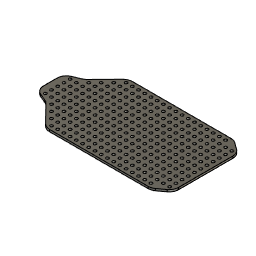
Base Plate (Autodesk Fusion 360 design; units mm, degrees)
Autodesk Fusion 360 part; units mm, degrees
sketch "Sketch1" plane through (0, 0, 0) normal (0, 0, 1) x (1, 0, 0)
  line L0 (-125, 0) -> (125, 0)
  line L1 (-125, 0) -> (-125, 21)
  line L2 (-125, 21) -> (-101, 31)
  line L3 (-101, 31) -> (-66, 66.7071)
  line L4 (-66, 66.7071) -> (104, 66.7071)
  line L5 (104, 66.7071) -> (125, 51.3774)
  line L6 (125, 51.3774) -> (125, 0)
  line L7 (-66, -66.7071) -> (104, -66.7071)
  line L8 (125, -51.3774) -> (125, 0)
  line L9 (-125, -21) -> (-101, -31)
  line L10 (104, -66.7071) -> (125, -51.3774)
  line L11 (-101, -31) -> (-66, -66.7071)
  line L12 (-125, 0) -> (-125, -21)
  line L13 (-125, 0) -> (125, 0) construction
  dimension "d1" = 250
  dimension "d2" = 21
  dimension "d3" = 26
  dimension "d4" = 24
  dimension "d5" = 50
  dimension "d6" = 35
  dimension "d7" = 170
  dimension "d8" = 26
  constraint horizontal L0
  constraint midpoint origin L0
  constraint perpendicular L0 L1
  constraint horizontal L4
  constraint symmetric L1.start L0 L12.start
  constraint symmetric L6.end L0 L8.end
  constraint symmetric L0 L1.end L9.start
  constraint symmetric L0 L2.end L9.end
  constraint symmetric L0 L3.end L7.start
  constraint symmetric L0 L4.end L7.end
  constraint symmetric L0 L5.end L8.start
  constraint vertical L6
  measures "d1" distance of L0.start L0.end
  measures "d2" distance of L0.start L1.end
  measures "d3" distance of L1.end L2.end
  measures "d4" horizontal distance of L1.end L2.end
  measures "d5" distance of L2.end L3.end
  measures "d6" horizontal distance of L2.end L3.end
  measures "d7" distance of L3.end L4.end
  measures "d8" distance of L4.end L5.end
extrude "Extrude1" add sketch "Sketch1" along normal blind 3.175
fillet "Fillet1" radius 15 10 edges at (-101, -31, 1.5875) (-125, -21, 1.5875) (-101, 31, 1.5875) (-125, 21, 1.5875) (-66, 66.7071, 1.5875) (-66, -66.7071, 1.5875) (104, -66.7071, 1.5875) (125, -51.3774, 1.5875) (125, 51.3774, 1.5875) (104, 66.7071, 1.5875)
sketch "Sketch2" plane through (0, 0, 3.175) normal (0, 0, 1) x (-1, 0, 0)
  arc A0 (-107.9516, -63.8225) -> (-99.1075, -66.7071) centre (-99.1075, -51.7071) ccw
  line L0 (-99.1075, -66.7071) -> (59.6987, -66.7071)
  arc A1 (59.6987, -66.7071) -> (70.4109, -62.2071) centre (59.6987, -51.7071) ccw
  line L1 (70.4109, -62.2071) -> (98.8682, -33.1748)
  arc A2 (103.8111, -29.8287) -> (98.8682, -33.1748) centre (109.5804, -43.6748) ccw
  line L2 (103.8111, -29.8287) -> (115.7692, -24.8462)
  arc A3 (115.7692, -24.8462) -> (125, -11) centre (110, -11) ccw
  line L3 (125, -11) -> (125, 11)
  arc A4 (125, 11) -> (115.7692, 24.8462) centre (110, 11) ccw
  line L4 (115.7692, 24.8462) -> (103.8111, 29.8287)
  arc A5 (98.8682, 33.1748) -> (103.8111, 29.8287) centre (109.5804, 43.6748) ccw
  line L5 (98.8682, 33.1748) -> (70.4109, 62.2071)
  arc A6 (70.4109, 62.2071) -> (59.6987, 66.7071) centre (59.6987, 51.7071) ccw
  line L6 (59.6987, 66.7071) -> (-99.1075, 66.7071)
  arc A7 (-99.1075, 66.7071) -> (-107.9516, 63.8225) centre (-99.1075, 51.7071) ccw
  line L7 (-107.9516, 63.8225) -> (-118.8441, 55.8712)
  arc A8 (-118.8441, 55.8712) -> (-125, 43.7558) centre (-110, 43.7558) ccw
  line L8 (-125, 43.7558) -> (-125, -43.7558)
  arc A9 (-125, -43.7558) -> (-118.8441, -55.8712) centre (-110, -43.7558) ccw
  line L9 (-118.8441, -55.8712) -> (-107.9516, -63.8225)
  circle A10 centre (-117, 0) radius 2.25
  line L10 (-125, 0) -> (125, 0) construction
  circle A11 centre (-117, 0) radius 2.25
  point P0 (-107, 0)
  point P1 (-97, 0)
  point P2 (-117, 10)
  point P3 (-107, 10)
  point P4 (-97, 10)
  point P5 (-117, 20)
  point P6 (-107, 20)
  point P7 (-97, 20)
  point P8 (-87, 0)
  point P9 (-77, 0)
  point P10 (-67, 0)
  point P11 (-57, 0)
  point P12 (-47, 0)
  point P13 (-37, 0)
  point P14 (-27, 0)
  point P15 (-17, 0)
  point P16 (-7, 0)
  point P17 (3, 0)
  point P18 (13, 0)
  point P19 (23, 0)
  point P20 (33, 0)
  point P21 (43, 0)
  point P22 (53, 0)
  point P23 (63, 0)
  point P24 (73, 0)
  point P25 (83, 0)
  point P26 (93, 0)
  point P27 (103, 0)
  point P28 (113, 0)
  point P29 (-87, 10)
  point P30 (-77, 10)
  point P31 (-67, 10)
  point P32 (-57, 10)
  point P33 (-47, 10)
  point P34 (-37, 10)
  point P35 (-27, 10)
  point P36 (-17, 10)
  point P37 (-7, 10)
  point P38 (3, 10)
  point P39 (13, 10)
  point P40 (23, 10)
  point P41 (33, 10)
  point P42 (43, 10)
  point P43 (53, 10)
  point P44 (63, 10)
  point P45 (73, 10)
  point P46 (83, 10)
  point P47 (93, 10)
  point P48 (103, 10)
  point P49 (113, 10)
  point P50 (-87, 20)
  point P51 (-77, 20)
  point P52 (-67, 20)
  point P53 (-57, 20)
  point P54 (-47, 20)
  point P55 (-37, 20)
  point P56 (-27, 20)
  point P57 (-17, 20)
  point P58 (-7, 20)
  point P59 (3, 20)
  point P60 (13, 20)
  point P61 (23, 20)
  point P62 (33, 20)
  point P63 (43, 20)
  point P64 (53, 20)
  point P65 (63, 20)
  point P66 (73, 20)
  point P67 (83, 20)
  point P68 (93, 20)
  point P69 (103, 20)
  point P70 (113, 20)
  point P71 (-117, 30)
  point P72 (-107, 30)
  point P73 (-97, 30)
  point P74 (-87, 30)
  point P75 (-77, 30)
  point P76 (-67, 30)
  point P77 (-57, 30)
  point P78 (-47, 30)
  point P79 (-37, 30)
  point P80 (-27, 30)
  point P81 (-17, 30)
  point P82 (-7, 30)
  point P83 (3, 30)
  point P84 (13, 30)
  point P85 (23, 30)
  point P86 (33, 30)
  point P87 (43, 30)
  point P88 (53, 30)
  point P89 (63, 30)
  point P90 (73, 30)
  point P91 (83, 30)
  point P92 (93, 30)
  point P93 (-117, 40)
  point P94 (-107, 40)
  point P95 (-97, 40)
  point P96 (-87, 40)
  point P97 (-77, 40)
  point P98 (-67, 40)
  point P99 (-57, 40)
  point P100 (-47, 40)
  point P101 (-37, 40)
  point P102 (-27, 40)
  point P103 (-17, 40)
  point P104 (-7, 40)
  point P105 (3, 40)
  point P106 (13, 40)
  point P107 (23, 40)
  point P108 (33, 40)
  point P109 (43, 40)
  point P110 (53, 40)
  point P111 (63, 40)
  point P112 (73, 40)
  point P113 (83, 40)
  point P114 (-117, 50)
  point P115 (-107, 50)
  point P116 (-97, 50)
  point P117 (-87, 50)
  point P118 (-77, 50)
  point P119 (-67, 50)
  point P120 (-57, 50)
  point P121 (-47, 50)
  point P122 (-37, 50)
  point P123 (-27, 50)
  point P124 (-17, 50)
  point P125 (-7, 50)
  point P126 (3, 50)
  point P127 (13, 50)
  point P128 (23, 50)
  point P129 (33, 50)
  point P130 (43, 50)
  point P131 (53, 50)
  point P132 (63, 50)
  point P133 (73, 50)
  point P134 (-97, 60)
  point P135 (-87, 60)
  point P136 (-77, 60)
  point P137 (-67, 60)
  point P138 (-57, 60)
  point P139 (-47, 60)
  point P140 (-37, 60)
  point P141 (-27, 60)
  point P142 (-17, 60)
  point P143 (-7, 60)
  point P144 (3, 60)
  point P145 (13, 60)
  point P146 (23, 60)
  point P147 (33, 60)
  point P148 (43, 60)
  point P149 (53, 60)
  point P150 (63, 60)
  point P151 (93, 0)
  point P152 (103, 0)
  point P153 (83, -10)
  point P154 (113, 0)
  point P155 (83, -20)
  point P156 (83, 0)
  point P157 (113, -10)
  point P158 (113, -20)
  point P159 (73, -20)
  point P160 (93, -10)
  point P161 (103, -20)
  point P162 (73, 0)
  point P163 (73, -10)
  point P164 (103, -10)
  point P165 (93, -20)
  point P166 (-67, -30)
  point P167 (-37, -40)
  point P168 (-47, -50)
  point P169 (-7, -10)
  point P170 (-117, -30)
  point P171 (3, -30)
  point P172 (-17, -50)
  point P173 (-47, -10)
  point P174 (-67, 0)
  point P175 (-107, -40)
  point P176 (-57, -40)
  point P177 (33, 0)
  point P178 (-107, -50)
  point P179 (-87, 0)
  point P180 (-117, -20)
  point P181 (-67, -50)
  point P182 (-57, -30)
  point P183 (-7, -50)
  point P184 (53, -30)
  point P185 (-47, -30)
  point P186 (-17, -40)
  point P187 (13, -10)
  point P188 (-107, -30)
  point P189 (-27, -20)
  point P190 (-77, -20)
  point P191 (-87, -10)
  point P192 (23, -20)
  point P193 (53, -20)
  point P194 (-47, -40)
  point P195 (-17, 0)
  point P196 (-27, -10)
  point P197 (-107, -10)
  point P198 (-27, -50)
  point P199 (-97, -40)
  point P200 (-37, -50)
  point P201 (-117, -10)
  point P202 (-7, -40)
  point P203 (63, -50)
  point P204 (63, -40)
  point P205 (-77, -30)
  point P206 (-87, -20)
  point P207 (-97, -20)
  point P208 (63, -10)
  point P209 (63, -30)
  point P210 (43, 0)
  point P211 (-7, -20)
  point P212 (3, 0)
  point P213 (63, -20)
  point P214 (63, 0)
  point P215 (-67, -20)
  point P216 (33, -30)
  point P217 (53, -10)
  point P218 (13, -40)
  point P219 (23, -30)
  point P220 (23, 0)
  point P221 (-87, -40)
  point P222 (-97, 0)
  point P223 (-107, 0)
  point P224 (-97, -30)
  point P225 (33, -20)
  point P226 (-107, -20)
  point P227 (-67, -10)
  point P228 (-77, 0)
  point P229 (-57, -50)
  point P230 (-7, -30)
  point P231 (-57, 0)
  point P232 (-77, -10)
  point P233 (-117, -50)
  point P234 (-27, -30)
  point P235 (-47, 0)
  point P236 (33, -10)
  point P237 (43, -20)
  point P238 (3, -10)
  point P239 (-97, -10)
  point P240 (53, -40)
  point P241 (23, -40)
  point P242 (33, -50)
  point P243 (23, -10)
  point P244 (43, -30)
  point P245 (3, -40)
  point P246 (-17, -10)
  point P247 (43, -40)
  point P248 (-77, -50)
  point P249 (-87, -50)
  point P250 (33, -40)
  point P251 (-27, 0)
  point P252 (13, -30)
  point P253 (-7, 0)
  point P254 (3, -50)
  point P255 (-77, -40)
  point P256 (-87, -30)
  point P257 (-17, -20)
  point P258 (13, -20)
  point P259 (-67, -40)
  point P260 (13, -50)
  point P261 (-27, -40)
  point P262 (-47, -20)
  point P263 (53, -50)
  point P264 (-97, -50)
  point P265 (23, -50)
  point P266 (-117, -40)
  point P267 (53, 0)
  point P268 (3, -20)
  point P269 (43, -50)
  point P270 (-37, -30)
  point P271 (13, 0)
  point P272 (43, -10)
  point P273 (-57, -10)
  point P274 (-57, -20)
  point P275 (-37, -10)
  point P276 (-37, 0)
  point P277 (-17, -30)
  point P278 (-37, -20)
  point P279 (73, -40)
  point P280 (83, -30)
  point P281 (73, -30)
  point P282 (73, -50)
  point P283 (83, -40)
  point P284 (93, -30)
  point P285 (-67, -60)
  point P286 (63, -60)
  point P287 (-17, -60)
  point P288 (13, -60)
  point P289 (43, -60)
  point P290 (-77, -60)
  point P291 (23, -60)
  point P292 (-97, -60)
  point P293 (3, -60)
  point P294 (33, -60)
  point P295 (-7, -60)
  point P296 (-57, -60)
  point P297 (-37, -60)
  point P298 (-27, -60)
  point P299 (-47, -60)
  point P300 (-87, -60)
  point P301 (53, -60)
  dimension "d14" = 4.5
  dimension "d15" = 8
  dimension "d18" = 10
  dimension "d19" = 10
  constraint midpoint L8 L10.start
  constraint midpoint L3 L10.end
  constraint symmetric A10 L10 A11
  constraint symmetric P223 L10 P0
  constraint symmetric P222 L10 P1
  constraint symmetric P2 L10 P201
  constraint symmetric P3 L10 P197
  constraint symmetric P4 L10 P239
  constraint symmetric P5 L10 P180
  constraint symmetric P6 L10 P226
  constraint symmetric P7 L10 P207
  constraint symmetric P179 L10 P8
  constraint symmetric P228 L10 P9
  constraint symmetric P174 L10 P10
  constraint symmetric P231 L10 P11
  constraint symmetric P235 L10 P12
  constraint symmetric P276 L10 P13
  constraint symmetric P251 L10 P14
  constraint symmetric P195 L10 P15
  constraint symmetric P253 L10 P16
  constraint symmetric P212 L10 P17
  constraint symmetric P271 L10 P18
  constraint symmetric P220 L10 P19
  constraint symmetric P177 L10 P20
  constraint symmetric P210 L10 P21
  constraint symmetric P267 L10 P22
  constraint symmetric P214 L10 P23
  constraint symmetric P162 L10 P24
  constraint symmetric P156 L10 P25
  constraint symmetric P151 L10 P26
  constraint symmetric P152 L10 P27
  constraint symmetric P154 L10 P28
  constraint symmetric P29 L10 P191
  constraint symmetric P30 L10 P232
  constraint symmetric P31 L10 P227
  constraint symmetric P32 L10 P273
  constraint symmetric P33 L10 P173
  constraint symmetric P34 L10 P275
  constraint symmetric P35 L10 P196
  constraint symmetric P36 L10 P246
  constraint symmetric P37 L10 P169
  constraint symmetric P38 L10 P238
  constraint symmetric P39 L10 P187
  constraint symmetric P40 L10 P243
  constraint symmetric P41 L10 P236
  constraint symmetric P42 L10 P272
  constraint symmetric P43 L10 P217
  constraint symmetric P44 L10 P208
  constraint symmetric P45 L10 P163
  constraint symmetric P46 L10 P153
  constraint symmetric P47 L10 P160
  constraint symmetric P48 L10 P164
  constraint symmetric P49 L10 P157
  constraint symmetric P50 L10 P206
  constraint symmetric P51 L10 P190
  constraint symmetric P52 L10 P215
  constraint symmetric P53 L10 P274
  constraint symmetric P54 L10 P262
  constraint symmetric P55 L10 P278
  constraint symmetric P56 L10 P189
  constraint symmetric P57 L10 P257
  constraint symmetric P58 L10 P211
  constraint symmetric P59 L10 P268
  constraint symmetric P60 L10 P258
  constraint symmetric P61 L10 P192
  constraint symmetric P62 L10 P225
  constraint symmetric P63 L10 P237
  constraint symmetric P64 L10 P193
  constraint symmetric P65 L10 P213
  constraint symmetric P66 L10 P159
  constraint symmetric P67 L10 P155
  constraint symmetric P68 L10 P165
  constraint symmetric P69 L10 P161
  constraint symmetric P70 L10 P158
  constraint symmetric P71 L10 P170
  constraint symmetric P72 L10 P188
  constraint symmetric P73 L10 P224
  constraint symmetric P74 L10 P256
  constraint symmetric P75 L10 P205
  constraint symmetric P76 L10 P166
  constraint symmetric P77 L10 P182
  constraint symmetric P78 L10 P185
  constraint symmetric P79 L10 P270
  constraint symmetric P80 L10 P234
  constraint symmetric P81 L10 P277
  constraint symmetric P82 L10 P230
  constraint symmetric P83 L10 P171
  constraint symmetric P84 L10 P252
  constraint symmetric P85 L10 P219
  constraint symmetric P86 L10 P216
  constraint symmetric P87 L10 P244
  constraint symmetric P88 L10 P184
  constraint symmetric P89 L10 P209
  constraint symmetric P90 L10 P281
  constraint symmetric P91 L10 P280
  constraint symmetric P92 L10 P284
  constraint symmetric P93 L10 P266
  constraint symmetric P94 L10 P175
  constraint symmetric P95 L10 P199
  constraint symmetric P96 L10 P221
  constraint symmetric P97 L10 P255
  constraint symmetric P98 L10 P259
  constraint symmetric P99 L10 P176
  constraint symmetric P100 L10 P194
  constraint symmetric P101 L10 P167
  constraint symmetric P102 L10 P261
  constraint symmetric P103 L10 P186
  constraint symmetric P104 L10 P202
  constraint symmetric P105 L10 P245
  constraint symmetric P106 L10 P218
  constraint symmetric P107 L10 P241
  constraint symmetric P108 L10 P250
  constraint symmetric P109 L10 P247
  constraint symmetric P110 L10 P240
  constraint symmetric P111 L10 P204
  constraint symmetric P112 L10 P279
  constraint symmetric P113 L10 P283
  constraint symmetric P114 L10 P233
  constraint symmetric P115 L10 P178
  constraint symmetric P116 L10 P264
  constraint symmetric P117 L10 P249
  constraint symmetric P118 L10 P248
  constraint symmetric P119 L10 P181
  constraint symmetric P120 L10 P229
  constraint symmetric P121 L10 P168
  constraint symmetric P122 L10 P200
  constraint symmetric P123 L10 P198
  constraint symmetric P124 L10 P172
  constraint symmetric P125 L10 P183
  constraint symmetric P126 L10 P254
  constraint symmetric P127 L10 P260
  constraint symmetric P128 L10 P265
  constraint symmetric P129 L10 P242
  constraint symmetric P130 L10 P269
  constraint symmetric P131 L10 P263
  constraint symmetric P132 L10 P203
  constraint symmetric P133 L10 P282
  constraint symmetric P134 L10 P292
  constraint symmetric P135 L10 P300
  constraint symmetric P136 L10 P290
  constraint symmetric P137 L10 P285
  constraint symmetric P138 L10 P296
  constraint symmetric P139 L10 P299
  constraint symmetric P140 L10 P297
  constraint symmetric P141 L10 P298
  constraint symmetric P142 L10 P287
  constraint symmetric P143 L10 P295
  constraint symmetric P144 L10 P293
  constraint symmetric P145 L10 P288
  constraint symmetric P146 L10 P291
  constraint symmetric P147 L10 P294
  constraint symmetric P148 L10 P289
  constraint symmetric P149 L10 P301
  constraint symmetric P150 L10 P286
  measures "d14" diameter of A10
  measures "d15" distance of L8 A10.centre
hole "Hole1" at (67, 20, 3.175) at (87, 50, 3.175) at (-43, -40, 3.175) at (17, 20, 3.175) at (-23, -50, 3.175) at (87, 30, 3.175) at (107, -40, 3.175) at (117, -50, 3.175) at (-13, -60, 3.175) at (-33, 20, 3.175) at (77, 40, 3.175) at (117, 20, 3.175) at (-73, -10, 3.175) at (47, 40, 3.175) at (-103, -20, 3.175) at (57, 30, 3.175) at (97, 50, 3.175) at (97, -50, 3.175) at (17, 30, 3.175) at (67, 40, 3.175) at (-53, 60, 3.175) at (67, -50, 3.175) at (-23, 50, 3.175) at (-53, -40, 3.175) at (97, 30, 3.175) at (97, 20, 3.175) at (57, 20, 3.175) at (117, 50, 3.175) at (-23, -60, 3.175) at (-83, -20, 3.175) at (27, 30, 3.175) at (-13, -50, 3.175) at (-43, 40, 3.175) at (-3, -50, 3.175) at (-3, -40, 3.175) at (87, 20, 3.175) at (77, 60, 3.175) at (-23, 40, 3.175) at (37, 30, 3.175) at (-73, -30, 3.175) at (-73, 20, 3.175) at (-113, 20, 3.175) at (77, -60, 3.175) at (47, 30, 3.175) at (97, -60, 3.175) at (77, -50, 3.175) at (77, 30, 3.175) at (-103, 0, 3.175) at (97, 40, 3.175) at (67, -60, 3.175) at (-93, 30, 3.175) at (7, 20, 3.175) at (-83, 30, 3.175) at (117, -40, 3.175) at (-43, -60, 3.175) at (7, 0, 3.175) at (107, -10, 3.175) at (7, -20, 3.175) at (57, -60, 3.175) at (7, -50, 3.175) at (117, 10, 3.175) at (117, 0, 3.175) at (37, -30, 3.175) at (-43, -30, 3.175) at (7, -60, 3.175) at (-3, 0, 3.175) at (-53, -20, 3.175) at (37, 0, 3.175) at (17, -60, 3.175) at (37, -40, 3.175) at (-53, 0, 3.175) at (7, 0, 3.175) at (107, -20, 3.175) at (107, 0, 3.175) at (27, -10, 3.175) at (87, -10, 3.175) at (-23, 10, 3.175) at (87, 10, 3.175) at (47, -40, 3.175) at (77, 0, 3.175) at (27, -50, 3.175) at (67, -30, 3.175) at (17, 0, 3.175) at (-3, 0, 3.175) at (107, 0, 3.175) at (57, -30, 3.175) at (-23, -10, 3.175) at (77, 10, 3.175) at (17, -50, 3.175) at (-33, -20, 3.175) at (7, -30, 3.175) at (17, 40, 3.175) at (57, 50, 3.175) at (-73, 50, 3.175) at (-83, 40, 3.175) at (-33, 30, 3.175) at (7, 60, 3.175) at (47, 20, 3.175) at (47, 50, 3.175) at (-33, 50, 3.175) at (-73, 30, 3.175) at (-63, 40, 3.175) at (-93, 10, 3.175) at (-13, -40, 3.175) at (-53, 40, 3.175) at (27, 60, 3.175) at (-43, 60, 3.175) at (-63, 60, 3.175) at (7, 30, 3.175) at (27, 50, 3.175) at (-53, 30, 3.175) at (37, 40, 3.175) at (-63, 50, 3.175) at (-43, -50, 3.175) at (47, 60, 3.175) at (67, 60, 3.175) at (67, 50, 3.175) at (17, 50, 3.175) at (107, 50, 3.175) at (-63, 20, 3.175) at (-33, -50, 3.175) at (7, 50, 3.175) at (-33, -40, 3.175) at (-3, 60, 3.175) at (57, 40, 3.175) at (17, 60, 3.175) at (-33, -60, 3.175) at (107, 30, 3.175) at (-23, -40, 3.175) at (-53, -50, 3.175) at (117, 40, 3.175) at (107, 40, 3.175) at (107, 20, 3.175) at (-53, -60, 3.175) at (-83, 20, 3.175) at (-3, 30, 3.175) at (-13, 40, 3.175) at (-3, -60, 3.175) at (-63, 10, 3.175) at (-13, 30, 3.175) at (77, 50, 3.175) at (77, 20, 3.175) at (87, 40, 3.175) at (-103, 20, 3.175) at (-103, 10, 3.175) at (-23, 20, 3.175) at (87, 60, 3.175) at (117, 30, 3.175) at (37, 50, 3.175) at (37, 60, 3.175) at (-3, 50, 3.175) at (7, 40, 3.175) at (-23, 30, 3.175) at (117, -20, 3.175) at (7, -40, 3.175) at (-63, 0, 3.175) at (87, 0, 3.175) at (87, -30, 3.175) at (-53, -10, 3.175) at (27, 0, 3.175) at (67, -20, 3.175) at (-93, 0, 3.175) at (-23, -30, 3.175) at (57, -20, 3.175) at (17, -20, 3.175) at (7, -10, 3.175) at (-43, 0, 3.175) at (17, -40, 3.175) at (57, -10, 3.175) at (27, -40, 3.175) at (47, -60, 3.175) at (-23, 0, 3.175) at (47, 10, 3.175) at (-13, 0, 3.175) at (97, 0, 3.175) at (47, -50, 3.175) at (-13, 0, 3.175) at (-33, 0, 3.175) at (57, -40, 3.175) at (27, -20, 3.175) at (-13, -10, 3.175) at (57, -50, 3.175) at (27, -60, 3.175) at (37, 0, 3.175) at (117, -30, 3.175) at (117, -10, 3.175) at (37, 10, 3.175) at (-3, -20, 3.175) at (17, 0, 3.175) at (-23, 0, 3.175) at (-93, 0, 3.175) at (97, 60, 3.175) at (107, -50, 3.175) at (67, 30, 3.175) at (-33, 10, 3.175) at (-83, 0, 3.175) at (-113, 0, 3.175) at (-103, 0, 3.175) at (7, 10, 3.175) at (-63, -10, 3.175) at (-113, -10, 3.175) at (-43, -10, 3.175) at (17, -30, 3.175) at (67, -40, 3.175) at (97, -40, 3.175) at (-113, -20, 3.175) at (-13, 10, 3.175) at (-73, -20, 3.175) at (87, -50, 3.175) at (27, 10, 3.175) at (-43, 10, 3.175) at (87, -40, 3.175) at (87, -60, 3.175) at (77, 0, 3.175) at (-23, -20, 3.175) at (117, 0, 3.175) at (-3, -10, 3.175) at (-13, -30, 3.175) at (57, 0, 3.175) at (97, -30, 3.175) at (37, -50, 3.175) at (77, -20, 3.175) at (37, -60, 3.175) at (47, -20, 3.175) at (57, 0, 3.175) at (-103, -10, 3.175) at (-53, 0, 3.175) at (-83, 0, 3.175) at (-73, 0, 3.175) at (-83, -40, 3.175) at (57, 10, 3.175) at (77, -40, 3.175) at (-73, -40, 3.175) at (-93, -20, 3.175) at (-63, 0, 3.175) at (-33, -30, 3.175) at (17, 10, 3.175) at (37, -20, 3.175) at (-43, -20, 3.175) at (27, 0, 3.175) at (-83, -30, 3.175) at (-63, -60, 3.175) at (77, -30, 3.175) at (-3, -30, 3.175) at (47, -30, 3.175) at (-53, -30, 3.175) at (47, -10, 3.175) at (-3, 10, 3.175) at (97, 0, 3.175) at (-113, 0, 3.175) at (107, 10, 3.175) at (27, -30, 3.175) at (-33, 0, 3.175) at (-63, -20, 3.175) at (-13, -20, 3.175) at (-73, -50, 3.175) at (-93, -10, 3.175) at (-93, -30, 3.175) at (-63, -50, 3.175) at (77, -10, 3.175) at (-63, -30, 3.175) at (-43, 0, 3.175) at (17, -10, 3.175) at (47, 0, 3.175) at (47, 0, 3.175) at (37, -10, 3.175) at (97, -10, 3.175) at (-73, 0, 3.175) at (-53, 10, 3.175) at (87, -20, 3.175) at (67, 0, 3.175) at (-83, -10, 3.175) at (-33, -10, 3.175) at (-63, -40, 3.175) at (67, -10, 3.175) at (67, 0, 3.175) at (97, 10, 3.175) at (97, -20, 3.175) at (87, 0, 3.175) at (67, 10, 3.175) at (107, -30, 3.175) at (-3, 20, 3.175) at (-33, 40, 3.175) at (-73, 10, 3.175) at (-23, 60, 3.175) at (-73, 40, 3.175) at (-53, 20, 3.175) at (-13, 60, 3.175) at (57, 60, 3.175) at (-43, 20, 3.175) at (-63, 30, 3.175) at (-43, 50, 3.175) at (-33, 60, 3.175) at (-53, 50, 3.175) at (-93, 20, 3.175) at (-13, 50, 3.175) at (-13, 20, 3.175) at (-83, 10, 3.175) at (27, 20, 3.175) at (-43, 30, 3.175) at (27, 40, 3.175) at (-113, 10, 3.175) at (-3, 40, 3.175) at (37, 20, 3.175) direction (0, 0, -1) diameter 4.5 depth 4 tip angle 118
equation "d2 = ( 42 / 2 ) * 1 mm"
